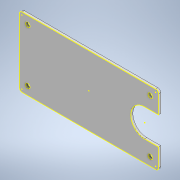
# Autodesk Inventor part: MCU_Power_PCB
Saved by Autodesk Inventor 2022 (Build 260153000, 153)
## iProperties
Created: 2021-11-05
Part Number: MCU_Power_PCB
Material: Generic
Document SubType Name: Modeling
Designer: Viktor
Density: 1 g/cm^3
Appearance: Default
Author: Viktor
Autodesk Inventor part; units mm, degrees
ref_plane "YZ Plane" through (0, 0, 0) normal (1, 0, 0) x (0, 1, 0)
ref_plane "XZ Plane" through (0, 0, 0) normal (0, 1, 0) x (-1, 0, 0)
ref_plane "XY Plane" through (0, 0, 0) normal (0, 0, 1) x (1, 0, 0)
sketch "Sketch1" plane through (0, 0, 0) normal (0, 0, 1) x (1, 0, 0)
  line L0 (-50, -25) -> (50, -25)
  line L1 (50, -25) -> (50, 25)
  line L2 (50, 25) -> (-50, 25)
  line L3 (-50, 25) -> (-50, -25)
  line L4 (-50, -25) -> (50, 25) construction
  line L5 (50, -25) -> (-50, 25) construction
  circle A0 centre (44, 19) radius 1.6
  line L6 (0, 35.5799) -> (0, -35.5799) projected
  line L7 (-70.5799, 0) -> (70.5799, 0) projected
  circle A1 centre (44, 19) radius 5 construction
  circle A2 centre (-44, 19) radius 1.6
  circle A3 centre (-44, 19) radius 5 construction
  circle A4 centre (44, -19) radius 1.6
  circle A5 centre (44, -19) radius 5 construction
  circle A6 centre (-44, -19) radius 1.6
  circle A7 centre (-44, -19) radius 5 construction
  circle A8 centre (40, 0) radius 10
  line L8 (40, 10) -> (50, 10)
  line L9 (40, -10) -> (50, -10)
  point P0 (0, 0)
  dimension "d0" = 100
  dimension "d1" = 50
  dimension "d2" = 6
  dimension "d3" = 6
  dimension "d4" = 3.2
  dimension "d5" = 10
  dimension "d9" = 20
  dimension "d10" = 10
  constraints: 16 end point, 9 centre point, 6 symmetric about line, 4 coincident, 3 parallel, 3 point on line, 2 midpoint, 2 perpendicular, 2 point on circle, 2 tangent, 1 horizontal, 6 other
  measures "d0" distance of L1.end L2.end
  measures "d1" distance of L0.end L1.end
  measures "d2" distance from line of L1 A0.centre
  measures "d3" distance from line of L2 A0.centre
  measures "d4" diameter of A0
  measures "d5" diameter of A1
  measures "d9" diameter of A8
  measures "d10" distance from line of L1 A8.centre
extrude "Extrusion1" add sketch "Sketch1" along normal blind 1.6 contours L3 L7 L6 L0 | L6 L7 A8 L9 L1 L0 | L3 L2 L6 L7 | L6 L2 L1 L8 A8 L7
fillet "Fillet1" radius 2 4 edges at (-50, 25, 0.8) (50, 25, 0.8) (50, -25, 0.8) (-50, -25, 0.8)
sketch "MCU_Power_PCB_Outline" plane through (0, 0, 1.6) normal (0, 0, 1) x (1, 0, 0)
  arc A0 (-50, -23) -> (-48, -25) centre (-48, -23) ccw projected
  line L0 (-48, -25) -> (48, -25) projected
  arc A1 (48, -25) -> (50, -23) centre (48, -23) ccw projected
  line L1 (50, -23) -> (50, -10) projected
  arc A2 (50, 23) -> (48, 25) centre (48, 23) ccw projected
  line L2 (48, 25) -> (-48, 25) projected
  arc A3 (-48, 25) -> (-50, 23) centre (-48, 23) ccw projected
  line L3 (-50, 23) -> (-50, -23) projected
  circle A4 centre (-44, -19) radius 1.6 projected
  circle A5 centre (44, -19) radius 1.6 projected
  circle A6 centre (44, 19) radius 1.6 projected
  circle A7 centre (-44, 19) radius 1.6 projected
  line L4 (50, -10) -> (40, -10) projected
  arc A8 (40, 10) -> (40, -10) centre (40, 0) ccw projected
  line L5 (40, 10) -> (50, 10) projected
  line L6 (50, 10) -> (50, 23) projected
  point P0 (0, 0)
equation "\"d3\" = d2"
body "Solid1"
